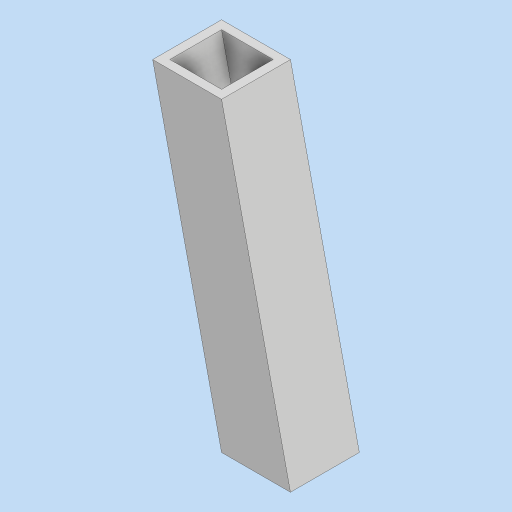
# Autodesk Inventor part: STRU_006_BilletPole_4.44in
Saved by Autodesk Inventor 2024.3 (Build 283343000, 343)
## iProperties
Created: 2024-07-23
Part Number: STRU_006_BilletPole_4.44in
Material: Generic
Document SubType Name: Modeling
Designer: bryan
Density: 1 g/cm^3
Appearance: Default
Author: bryan
Autodesk Inventor part; units mm, degrees
ref_plane "YZ Plane" through (0, 0, 0) normal (1, 0, 0) x (0, 1, 0)
ref_plane "XY Plane" through (0, 0, 0) normal (0, 0, 1) x (1, 0, 0)
sketch "Sketch1" plane through (0, 0, 0) normal (0, 1, 0) x (-1, 0, 0)
  line L0 (-12.7, -12.7) -> (12.7, -12.7)
  line L1 (12.7, -12.7) -> (12.7, 12.7)
  line L2 (12.7, 12.7) -> (-12.7, 12.7)
  line L3 (-12.7, 12.7) -> (-12.7, -12.7)
  line L4 (-12.7, -12.7) -> (12.7, 12.7) construction
  line L5 (12.7, -12.7) -> (-12.7, 12.7) construction
  line L6 (9.525, 9.525) -> (9.525, -9.525)
  line L7 (9.525, -9.525) -> (-9.525, -9.525)
  line L8 (-9.525, -9.525) -> (-9.525, 9.525)
  line L9 (-9.525, 9.525) -> (9.525, 9.525)
  point P0 (0, 0)
  dimension "d0" = 25.4
  dimension "d1" = 25.4
  dimension "d2" = 3.175
  constraints: 20 end point, 4 parallel, 2 midpoint, 2 perpendicular, 1 horizontal, 3 other
  measures "d0" distance of L2.end L1.end
  measures "d1" distance of L1.end L0.end
  measures "d2" distance between parallel lines of L1 L6
ref_plane "Work Plane1" through (0, 112.776, 0) normal (0, 1, 0) x (-1, 0, 0)
sketch "Sketch2" plane through (0, 112.776, 0) normal (0, 1, 0) x (-1, 0, 0)
  line L0 (38.1, -12.7) -> (12.7, -12.7)
  line L1 (12.7, -12.7) -> (12.7, 12.7)
  line L2 (12.7, 12.7) -> (38.1, 12.7)
  line L3 (38.1, 12.7) -> (38.1, -12.7)
  line L4 (38.1, -12.7) -> (12.7, 12.7) construction
  line L5 (12.7, -12.7) -> (38.1, 12.7) construction
  line L6 (34.925, 9.525) -> (15.875, 9.525)
  line L7 (15.875, 9.525) -> (15.875, -9.525)
  line L8 (15.875, -9.525) -> (34.925, -9.525)
  line L9 (34.925, -9.525) -> (34.925, 9.525)
  point P0 (0, 0)
  point P1 (25.4, 0)
  point P2 (38.1, 0)
  dimension "d6" = 25.4
  dimension "d7" = 25.4
  dimension "d8" = 3.175
  constraints: 20 end point, 4 parallel, 3 midpoint, 2 perpendicular, 1 coincident, 1 horizontal, 3 other
  measures "d6" distance of L1.end L2.end
  measures "d7" distance of L0.end L1.end
  measures "d8" distance from line of point (38.1, 0) L9
sketch "Sketch3" plane through (0, 0, 0) normal (0, 0, 1) x (1, 0, 0)
  line L0 (-12.7, 112.776) -> (-38.1, 112.776) construction
  line L1 (-25.4, 112.776) -> (0, 0)
  constraints: 2 end point, 1 midpoint
sweep "Sweep1" add profiles "Sketch1" path "Sketch3"
body "Solid2"
